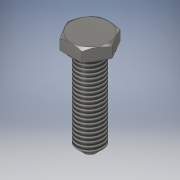
# Autodesk Inventor part: Door Hinge Pin
Saved by Autodesk Inventor 2018 (Build 220112000, 112)
## iProperties
Created: 2016-10-27
Part Number: Door Hinge Pin
Material: Steel, Carbon
Document SubType Name: Modeling
Designer: Joey
Density: 7.85 g/cm^3
Appearance: Semi-Polished
Mass: 8.75551 g
Surface Area: 8.6781 cm^2
Volume: 1.11535 cm^3
Author: Joey
Autodesk Inventor part; units mm, degrees
ref_plane "YZ Plane" through (0, 0, 0) normal (1, 0, 0) x (0, 1, 0)
ref_plane "XZ Plane" through (0, 0, 0) normal (0, 1, 0) x (-1, 0, 0)
ref_plane "XY Plane" through (0, 0, 0) normal (0, 0, 1) x (1, 0, 0)
sketch "Sketch1" plane through (0, 0, 0) normal (0, 0, 1) x (1, 0, 0)
  line L0 (0, 0) -> (6.35, 0)
  line L1 (6.35, 0) -> (6.35, -44.45)
  line L2 (6.35, -44.45) -> (0, -44.45)
  line L3 (0, -44.45) -> (0, 0)
  dimension "d0" = 12.7
  dimension "d1" = 44.45
  constraints: 8 end point, 2 parallel, 1 horizontal, 1 perpendicular
  measures "d0" diameter of L1 L3
  measures "d1" distance of L2.end L0.start
revolve "Revolution1" add sketch "Sketch1" angle 360 about axis through (0, -44.45, 0) along (0, 1, 0)
chamfer "Chamfer1" distance 3.175 angle 45 1 edges at (-6.35, -44.45, 0)
sketch "Sketch2" plane through (0, 0, 0) normal (0, 1, 0) x (1, 0, 0)
  circle A0 centre (0, 0) radius 9.525
  point P0 (0, 0)
  dimension "d6" = 19.05
  constraints: 1 centre point, 1 coincident
  measures "d6" diameter of A0
extrude "Extrusion1" add sketch "Sketch2" along normal blind 6.35
sketch "Sketch3" plane through (0, 6.35, 0) normal (0, 1, 0) x (1, 0, 0)
  line L0 (10.9985, 0) -> (5.4993, -9.525)
  line L1 (5.4993, -9.525) -> (-5.4993, -9.525)
  line L2 (-5.4993, -9.525) -> (-10.9985, 0)
  line L3 (-10.9985, 0) -> (-5.4993, 9.525)
  line L4 (-5.4993, 9.525) -> (5.4993, 9.525)
  line L5 (5.4993, 9.525) -> (10.9985, 0)
  circle A0 centre (0, 0) radius 9.525 construction
  point P0 (0, 0)
  point P1 (0, 0)
  constraints: 12 end point, 1 coincident, 1 horizontal, 1 tangent, 13 other
extrude "Extrusion2" add sketch "Sketch3" against normal blind 5.969
sketch "Sketch4" plane through (0, 0, 0) normal (0, 0, 1) x (1, 0, 0)
  line L0 (9.2388, 6.35) -> (10.9985, 6.35)
  line L1 (10.9985, 6.35) -> (10.9985, 5.334)
  line L2 (10.9985, 5.334) -> (9.2388, 6.35)
  line L3 (0, -1.5875) -> (0, 9.525) projected
  line L4 (5.4993, 0) -> (10.9985, 0) construction
  line L5 (5.4993, 6.35) -> (10.9985, 6.35) construction
  line L6 (5.4993, 6.35) -> (5.4993, 0.381) construction
  line L7 (10.9985, 6.35) -> (10.9985, 0.381) construction
  line L8 (10.9985, 6.35) -> (5.4993, 6.35) projected
  line L9 (8.2489, 0.381) -> (10.9985, 0.381) projected
  line L10 (5.4993, 0.381) -> (8.2489, 0.381) projected
  point P0 (0, 0)
  point P1 (16.2522, 7.9375)
  dimension "d11" = 30
  dimension "d17" = 1.016
  constraints: 6 end point, 2 collinear, 1 horizontal, 1 perpendicular
  measures "d11" angle of L2 L0
  measures "d17" distance of L0.end L1.end
revolve "Revolution2" cut sketch "Sketch4" angle 360 about axis through (0, -10, 0) along (0, 1, 0)
thread "Thread3" size "1/2-13 UNC" class "2A" standard "ANSI Unified Screw Threads" full length
equation "\"diameter\" = 1.8542"
equation "\"length\" = 19.05"
body "Solid1"
